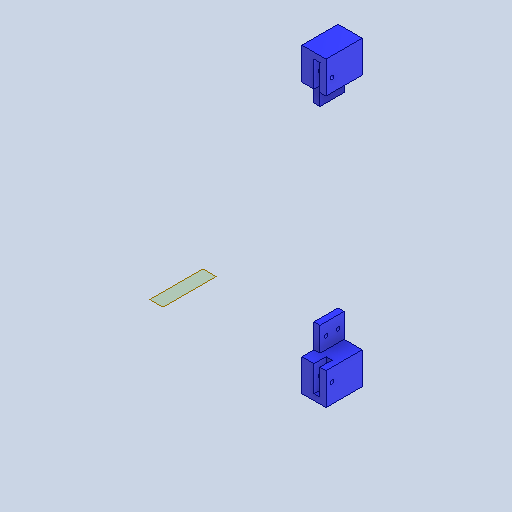
# Autodesk Inventor part: base_weel-v3-3DP-2
Saved by Autodesk Inventor 2025.2 (Build 292293000, 293)
## iProperties
Created: 2025-04-04
Part Number: base_weel-v3-3DP-2
Material: ABS プラスチック
Document SubType Name: Modeling
Designer: haruy
Density: 1.06 g/cm^3
Appearance: 青 - 壁塗料 - 光沢
Author: haruy
Autodesk Inventor part; units mm, degrees
ref_plane "YZ Plane" through (0, 0, 0) normal (1, 0, 0) x (0, 1, 0)
ref_plane "XZ Plane" through (0, 0, 0) normal (0, 1, 0) x (-1, 0, 0)
ref_plane "XY Plane" through (0, 0, 0) normal (0, 0, 1) x (1, 0, 0)
derived "base_weel-v3-3DP-1.ipt"
sketch "スケッチ1" plane through (0, 0, 0) normal (1, 0, 0) x (0, 1, 0)
  circle A0 centre (0, 0) radius 385
  circle A1 centre (0, 0) radius 360
  line L0 (190, 300) -> (-190, 300)
  line L1 (-190, 300) -> (-190, 280)
  line L2 (-190, 280) -> (190, 280)
  line L3 (190, 280) -> (190, 300)
  line L4 (300, 190) -> (280, 190)
  line L5 (280, 190) -> (280, -190)
  line L6 (280, -190) -> (300, -190)
  line L7 (300, -190) -> (300, 190)
  line L8 (208.9645, 286.7462) -> (286.7462, 208.9645)
  line L9 (286.7462, 208.9645) -> (272.6041, 194.8223)
  line L10 (272.6041, 194.8223) -> (194.8223, 272.6041)
  line L11 (194.8223, 272.6041) -> (208.9645, 286.7462)
  line L12 (208.9645, 286.7462) -> (318.9645, 286.7462) construction
  line L13 (118.4548, 217.4497) -> (217.4497, 118.4548)
  line L14 (217.4497, 118.4548) -> (203.3076, 104.3127)
  line L15 (203.3076, 104.3127) -> (104.3127, 203.3076)
  line L16 (104.3127, 203.3076) -> (118.4548, 217.4497)
  line L17 (118.4548, 217.4497) -> (258.4548, 217.4497) construction
  line L18 (189.519, 263.7652) -> (263.7652, 189.519)
  line L19 (263.7652, 189.519) -> (235.481, 161.2348)
  line L20 (235.481, 161.2348) -> (161.2348, 235.481)
  line L21 (161.2348, 235.481) -> (189.519, 263.7652)
  line L22 (189.519, 263.7652) -> (294.519, 263.7652) construction
  line L23 (180.6802, 201.8934) -> (201.8934, 180.6802)
  line L24 (201.8934, 180.6802) -> (194.8223, 173.6091)
  line L25 (194.8223, 173.6091) -> (173.6091, 194.8223)
  line L26 (173.6091, 194.8223) -> (180.6802, 201.8934)
  line L27 (180.6802, 201.8934) -> (210.6802, 201.8934) construction
  line L28 (170.0736, 198.3579) -> (198.3579, 170.0736)
  line L29 (198.3579, 170.0736) -> (194.1152, 165.831)
  line L30 (194.1152, 165.831) -> (165.831, 194.1152)
  line L31 (165.831, 194.1152) -> (170.0736, 198.3579)
  line L32 (198.3579, 170.0736) -> (194.1152, 165.831)
  line L33 (194.1152, 165.831) -> (222.3995, 137.5467)
  line L34 (222.3995, 137.5467) -> (226.6421, 141.7893)
  line L35 (226.6421, 141.7893) -> (198.3579, 170.0736)
  line L36 (197.6508, 162.2954) -> (218.864, 141.0822)
  line L37 (218.864, 141.0822) -> (211.7929, 134.0111)
  line L38 (211.7929, 134.0111) -> (190.5797, 155.2244)
  line L39 (190.5797, 155.2244) -> (197.6508, 162.2954)
  line L40 (182.448, 153.4566) -> (215.682, 120.2226)
  line L41 (215.682, 120.2226) -> (146.032, 50.5725)
  line L42 (146.032, 50.5725) -> (112.7979, 83.8066)
  line L43 (112.7979, 83.8066) -> (182.448, 153.4566)
  line L44 (193.4081, 142.4964) -> (199.065, 136.8396)
  line L45 (199.065, 136.8396) -> (215.5406, 153.3152)
  line L46 (215.5406, 153.3152) -> (209.8837, 158.972)
  line L47 (209.8837, 158.972) -> (193.4081, 142.4964)
  line L48 (58.5, 280) -> (38.5, 280)
  line L49 (38.5, 280) -> (38.5, -280)
  line L50 (38.5, -280) -> (58.5, -280)
  line L51 (58.5, -280) -> (58.5, 280)
  line L52 (280, 98.5) -> (58.5, 98.5)
  line L53 (58.5, 98.5) -> (58.5, 78.5)
  line L54 (58.5, 78.5) -> (280, 78.5)
  line L55 (280, 78.5) -> (280, 98.5)
  line L56 (156.5, 23.5) -> (58.5, 23.5)
  line L57 (58.5, 23.5) -> (58.5, -23.5)
  line L58 (58.5, -23.5) -> (156.5, -23.5)
  line L59 (156.5, -23.5) -> (156.5, 23.5)
  line L60 (98.5, 280) -> (78.5, 280)
  line L61 (78.5, 280) -> (78.5, 98.5)
  line L62 (78.5, 98.5) -> (98.5, 98.5)
  line L63 (98.5, 98.5) -> (98.5, 280)
  line L64 (23.5, 166.5) -> (-23.5, 166.5)
  line L65 (-23.5, 166.5) -> (-23.5, 68.5)
  line L66 (-23.5, 68.5) -> (23.5, 68.5)
  line L67 (23.5, 68.5) -> (23.5, 166.5)
  line L68 (-38.5, 280) -> (-58.5, 280)
  line L69 (-58.5, 280) -> (-58.5, -280)
  line L70 (-58.5, -280) -> (-38.5, -280)
  line L71 (-38.5, -280) -> (-38.5, 280)
  line L72 (23.5, -68.5) -> (-23.5, -68.5)
  line L73 (-23.5, -68.5) -> (-23.5, -166.5)
  line L74 (-23.5, -166.5) -> (23.5, -166.5)
  line L75 (23.5, -166.5) -> (23.5, -68.5)
  line L76 (-58.5, 23.5) -> (-156.5, 23.5)
  line L77 (-156.5, 23.5) -> (-156.5, -23.5)
  line L78 (-156.5, -23.5) -> (-58.5, -23.5)
  line L79 (-58.5, -23.5) -> (-58.5, 23.5)
  line L80 (-254.5584, -254.5584) -> (254.5584, -254.5584) construction
  line L81 (254.5584, -254.5584) -> (254.5584, 254.5584) construction
  line L82 (254.5584, 254.5584) -> (-254.5584, 254.5584) construction
  line L83 (-254.5584, 254.5584) -> (-254.5584, -254.5584) construction
  line L84 (-254.5584, -254.5584) -> (254.5584, 254.5584) construction
  line L85 (254.5584, -254.5584) -> (-254.5584, 254.5584) construction
  line L86 (254.5584, 254.5584) -> (0, 0)
  line L87 (0, 0) -> (0, 254.5584)
  line L88 (175.3769, 249.6231) -> (249.6231, 175.3769)
  line L89 (-212.5, -212.5) -> (212.5, -212.5) construction
  line L90 (212.5, -212.5) -> (212.5, 212.5) construction
  line L91 (212.5, 212.5) -> (-212.5, 212.5) construction
  line L92 (-212.5, 212.5) -> (-212.5, -212.5) construction
  line L93 (-212.5, -212.5) -> (212.5, 212.5) construction
  line L94 (212.5, -212.5) -> (-212.5, 212.5) construction
  line L95 (58.5, 68.5) -> (-58.5, 68.5)
  line L96 (-58.5, 68.5) -> (-58.5, 48.5)
  line L97 (-58.5, 48.5) -> (58.5, 48.5)
  line L98 (58.5, 48.5) -> (58.5, 68.5)
  line L99 (-58.5, -48.5) -> (58.5, -48.5)
  line L100 (58.5, -48.5) -> (58.5, -68.5)
  line L101 (58.5, -68.5) -> (-58.5, -68.5)
  line L102 (-58.5, -68.5) -> (-58.5, -48.5)
  line L103 (0, 0) -> (0, 300)
  line L104 (0, 0) -> (300, 0)
  line L105 (190, -300) -> (-190, -300)
  line L106 (-190, -300) -> (-190, -280)
  line L107 (-190, -280) -> (190, -280)
  line L108 (190, -280) -> (190, -300)
  line L109 (280, -98.5) -> (58.5, -98.5)
  line L110 (58.5, -78.5) -> (280, -78.5)
  line L111 (78.5, -280) -> (78.5, -98.5)
  line L112 (98.5, -98.5) -> (98.5, -280)
  line L113 (208.9645, -286.7462) -> (286.7462, -208.9645)
  line L114 (286.7462, -208.9645) -> (272.6041, -194.8223)
  line L115 (272.6041, -194.8223) -> (194.8223, -272.6041)
  line L116 (194.8223, -272.6041) -> (208.9645, -286.7462)
  line L117 (118.4548, -217.4497) -> (217.4497, -118.4548)
  line L118 (217.4497, -118.4548) -> (203.3076, -104.3127)
  line L119 (203.3076, -104.3127) -> (104.3127, -203.3076)
  line L120 (104.3127, -203.3076) -> (118.4548, -217.4497)
  line L121 (-300, 190) -> (-280, 190)
  line L122 (-280, 190) -> (-280, -190)
  line L123 (-280, -190) -> (-300, -190)
  line L124 (-300, -190) -> (-300, 190)
  line L125 (-208.9645, 286.7462) -> (-286.7462, 208.9645)
  line L126 (-286.7462, 208.9645) -> (-272.6041, 194.8223)
  line L127 (-272.6041, 194.8223) -> (-194.8223, 272.6041)
  line L128 (-194.8223, 272.6041) -> (-208.9645, 286.7462)
  line L129 (-118.4548, 217.4497) -> (-217.4497, 118.4548)
  line L130 (-217.4497, 118.4548) -> (-203.3076, 104.3127)
  line L131 (-203.3076, 104.3127) -> (-104.3127, 203.3076)
  line L132 (-104.3127, 203.3076) -> (-118.4548, 217.4497)
  line L133 (-280, 98.5) -> (-58.5, 98.5)
  line L134 (-58.5, 78.5) -> (-280, 78.5)
  line L135 (-78.5, 280) -> (-78.5, 98.5)
  line L136 (-98.5, 98.5) -> (-98.5, 280)
  line L137 (-98.5, -98.5) -> (-98.5, -280)
  line L138 (-78.5, -280) -> (-78.5, -98.5)
  line L139 (-280, -98.5) -> (-58.5, -98.5)
  line L140 (-58.5, -78.5) -> (-280, -78.5)
  line L141 (-208.9645, -286.7462) -> (-286.7462, -208.9645)
  line L142 (-194.8223, -272.6041) -> (-208.9645, -286.7462)
  line L143 (-272.6041, -194.8223) -> (-194.8223, -272.6041)
  line L144 (-286.7462, -208.9645) -> (-272.6041, -194.8223)
  line L145 (-118.4548, -217.4497) -> (-217.4497, -118.4548)
  line L146 (-104.3127, -203.3076) -> (-118.4548, -217.4497)
  line L147 (-203.3076, -104.3127) -> (-104.3127, -203.3076)
  line L148 (-217.4497, -118.4548) -> (-203.3076, -104.3127)
  line L149 (170, 300) -> (170, 280)
  line L150 (223.1066, 272.6041) -> (208.9645, 258.4619)
  circle A2 centre (175, 290) radius 1.6
  circle A3 centre (185, 290) radius 1.6
  circle A4 centre (205.4289, 276.1396) radius 1.6
  circle A5 centre (212.5, 269.0685) radius 1.6
  circle A6 centre (290, 175) radius 1.6
  circle A7 centre (290, 185) radius 1.6
  circle A8 centre (276.1396, 205.4289) radius 1.6
  circle A9 centre (269.0685, 212.5) radius 1.6
  line L151 (132.5969, 203.3076) -> (118.4548, 189.1655)
  line L152 (118.4548, 217.4497) -> (98.5, 237.4045)
  line L153 (104.3127, 203.3076) -> (98.5, 209.1203)
  line L154 (98.5, 209.1203) -> (78.5, 209.1203)
  circle A10 centre (88.5, 218) radius 1.6
  circle A11 centre (88.5, 228) radius 1.6
  line L155 (98.5, 237.4045) -> (78.5, 237.4045)
  circle A12 centre (121.9903, 199.7721) radius 1.6
  circle A13 centre (114.9193, 206.8431) radius 1.6
  circle A14 centre (218, 88.5) radius 1.6
  circle A15 centre (228, 88.5) radius 1.6
  circle A16 centre (199.7721, 121.9903) radius 1.6
  circle A17 centre (206.8431, 114.9193) radius 1.6
  line L156 (38.5, 280) -> (38.5, 300)
  line L157 (98.5, 280) -> (98.5, 300)
  line L158 (58.5, 260) -> (38.5, 260)
  line L159 (78.5, 260) -> (98.5, 260)
  circle A18 centre (88.5, 275) radius 1.6
  circle A19 centre (88.5, 265) radius 1.6
  circle A20 centre (48.5, 275) radius 1.6
  circle A21 centre (48.5, 265) radius 1.6
  circle A22 centre (88.5, 290) radius 1.6
  circle A23 centre (68.5, 290) radius 1.6
  circle A24 centre (48.5, 290) radius 1.6
  line L160 (260, 98.5) -> (260, 78.5)
  line L161 (300, 98.5) -> (280, 98.5)
  line L162 (280, 78.5) -> (300, 78.5)
  circle A25 centre (290, 78.5) radius 1.6
  circle A26 centre (290, 88.5) radius 1.6
  circle A27 centre (275, 88.5) radius 1.6
  circle A28 centre (265, 88.5) radius 1.6
  line L163 (78.5, 189.25) -> (58.5, 189.25)
  circle A29 centre (88.5, 103.5) radius 1.6
  circle A30 centre (88.5, 113.5) radius 1.6
  circle A31 centre (48.5, 103.5) radius 1.6
  circle A32 centre (48.5, 113.5) radius 1.6
  circle A33 centre (88.5, 88.5) radius 1.6
  circle A34 centre (68.5, 88.5) radius 1.6
  circle A35 centre (48.5, 88.5) radius 1.6
  circle A36 centre (48.5, 58.5) radius 1.6
  circle A37 centre (175, -290) radius 1.6
  circle A38 centre (185, -290) radius 1.6
  circle A39 centre (205.4289, -276.1396) radius 1.6
  circle A40 centre (212.5, -269.0685) radius 1.6
  circle A41 centre (276.1396, -205.4289) radius 1.6
  circle A42 centre (269.0685, -212.5) radius 1.6
  circle A43 centre (290, -185) radius 1.6
  circle A44 centre (290, -175) radius 1.6
  circle A45 centre (88.5, -218) radius 1.6
  circle A46 centre (88.5, -228) radius 1.6
  circle A47 centre (121.9903, -199.7721) radius 1.6
  circle A48 centre (114.9193, -206.8431) radius 1.6
  circle A49 centre (228, -88.5) radius 1.6
  circle A50 centre (218, -88.5) radius 1.6
  circle A51 centre (206.8431, -114.9193) radius 1.6
  circle A52 centre (199.7721, -121.9903) radius 1.6
  circle A53 centre (88.5, -275) radius 1.6
  circle A54 centre (88.5, -265) radius 1.6
  circle A55 centre (48.5, -275) radius 1.6
  circle A56 centre (48.5, -265) radius 1.6
  circle A57 centre (88.5, -290) radius 1.6
  circle A58 centre (68.5, -290) radius 1.6
  circle A59 centre (48.5, -290) radius 1.6
  circle A60 centre (290, -78.5) radius 1.6
  circle A61 centre (290, -88.5) radius 1.6
  circle A62 centre (275, -88.5) radius 1.6
  circle A63 centre (265, -88.5) radius 1.6
  circle A64 centre (88.5, -88.5) radius 1.6
  circle A65 centre (68.5, -88.5) radius 1.6
  circle A66 centre (48.5, -88.5) radius 1.6
  circle A67 centre (48.5, -103.5) radius 1.6
  circle A68 centre (48.5, -113.5) radius 1.6
  circle A69 centre (88.5, -103.5) radius 1.6
  circle A70 centre (88.5, -113.5) radius 1.6
  circle A71 centre (48.5, -58.5) radius 1.6
  circle A72 centre (-175, 290) radius 1.6
  circle A73 centre (-185, 290) radius 1.6
  circle A74 centre (-205.4289, 276.1396) radius 1.6
  circle A75 centre (-212.5, 269.0685) radius 1.6
  circle A76 centre (-276.1396, 205.4289) radius 1.6
  circle A77 centre (-269.0685, 212.5) radius 1.6
  circle A78 centre (-290, 185) radius 1.6
  circle A79 centre (-290, 175) radius 1.6
  circle A80 centre (-88.5, 218) radius 1.6
  circle A81 centre (-88.5, 228) radius 1.6
  circle A82 centre (-121.9903, 199.7721) radius 1.6
  circle A83 centre (-114.9193, 206.8431) radius 1.6
  circle A84 centre (-228, 88.5) radius 1.6
  circle A85 centre (-218, 88.5) radius 1.6
  circle A86 centre (-206.8431, 114.9193) radius 1.6
  circle A87 centre (-199.7721, 121.9903) radius 1.6
  circle A88 centre (-88.5, 275) radius 1.6
  circle A89 centre (-88.5, 265) radius 1.6
  circle A90 centre (-48.5, 275) radius 1.6
  circle A91 centre (-48.5, 265) radius 1.6
  circle A92 centre (-88.5, 290) radius 1.6
  circle A93 centre (-68.5, 290) radius 1.6
  circle A94 centre (-48.5, 290) radius 1.6
  circle A95 centre (-290, 78.5) radius 1.6
  circle A96 centre (-290, 88.5) radius 1.6
  circle A97 centre (-275, 88.5) radius 1.6
  circle A98 centre (-265, 88.5) radius 1.6
  circle A99 centre (-88.5, 88.5) radius 1.6
  circle A100 centre (-68.5, 88.5) radius 1.6
  circle A101 centre (-48.5, 88.5) radius 1.6
  circle A102 centre (-48.5, 103.5) radius 1.6
  circle A103 centre (-48.5, 113.5) radius 1.6
  circle A104 centre (-88.5, 103.5) radius 1.6
  circle A105 centre (-88.5, 113.5) radius 1.6
  circle A106 centre (-48.5, 58.5) radius 1.6
  circle A107 centre (-175, -290) radius 1.6
  circle A108 centre (-185, -290) radius 1.6
  circle A109 centre (-212.5, -269.0685) radius 1.6
  circle A110 centre (-205.4289, -276.1396) radius 1.6
  circle A111 centre (-269.0685, -212.5) radius 1.6
  circle A112 centre (-276.1396, -205.4289) radius 1.6
  circle A113 centre (-290, -185) radius 1.6
  circle A114 centre (-290, -175) radius 1.6
  circle A115 centre (-88.5, -290) radius 1.6
  circle A116 centre (-88.5, -275) radius 1.6
  circle A117 centre (-88.5, -265) radius 1.6
  circle A118 centre (-68.5, -290) radius 1.6
  circle A119 centre (-48.5, -290) radius 1.6
  circle A120 centre (-48.5, -275) radius 1.6
  circle A121 centre (-48.5, -265) radius 1.6
  circle A122 centre (-88.5, -228) radius 1.6
  circle A123 centre (-88.5, -218) radius 1.6
  circle A124 centre (-114.9193, -206.8431) radius 1.6
  circle A125 centre (-121.9903, -199.7721) radius 1.6
  circle A126 centre (-88.5, -113.5) radius 1.6
  circle A127 centre (-88.5, -103.5) radius 1.6
  circle A128 centre (-88.5, -88.5) radius 1.6
  circle A129 centre (-68.5, -88.5) radius 1.6
  circle A130 centre (-48.5, -88.5) radius 1.6
  circle A131 centre (-48.5, -103.5) radius 1.6
  circle A132 centre (-48.5, -113.5) radius 1.6
  circle A133 centre (-48.5, -58.5) radius 1.6
  circle A134 centre (-199.7721, -121.9903) radius 1.6
  circle A135 centre (-206.8431, -114.9193) radius 1.6
  circle A136 centre (-218, -88.5) radius 1.6
  circle A137 centre (-228, -88.5) radius 1.6
  circle A138 centre (-265, -88.5) radius 1.6
  circle A139 centre (-275, -88.5) radius 1.6
  circle A140 centre (-290, -78.5) radius 1.6
  circle A141 centre (-290, -88.5) radius 1.6
  line L164 (120, 280) -> (-120, 280)
  line L165 (-120, 280) -> (-120, 171.5)
  line L166 (-120, 171.5) -> (120, 171.5)
  line L167 (120, 171.5) -> (120, 280)
  line L168 (105, 300) -> (125, 300)
  line L169 (125, 300) -> (125, 280)
  line L170 (125, 280) -> (105, 280)
  line L171 (105, 280) -> (105, 300)
  line L172 (78.5, 171.5) -> (98.5, 171.5)
  line L173 (98.5, 171.5) -> (98.5, 151.5)
  line L174 (98.5, 151.5) -> (78.5, 151.5)
  line L175 (78.5, 151.5) -> (78.5, 171.5)
  circle A142 centre (120, 290) radius 1.6
  circle A143 centre (110, 290) radius 1.6
  circle A144 centre (88.5, 166.5) radius 1.6
  circle A145 centre (88.5, 156.5) radius 1.6
  circle A146 centre (-120, 290) radius 1.6
  circle A147 centre (-110, 290) radius 1.6
  circle A148 centre (-88.5, 166.5) radius 1.6
  circle A149 centre (-88.5, 156.5) radius 1.6
  circle A150 centre (120, -290) radius 1.6
  circle A151 centre (110, -290) radius 1.6
  circle A152 centre (88.5, -166.5) radius 1.6
  circle A153 centre (88.5, -156.5) radius 1.6
  circle A154 centre (-120, -290) radius 1.6
  circle A155 centre (-110, -290) radius 1.6
  circle A156 centre (-88.5, -166.5) radius 1.6
  circle A157 centre (-88.5, -156.5) radius 1.6
  line L176 (300, 73.5) -> (280, 73.5)
  circle A158 centre (290, 120) radius 1.6
  circle A159 centre (290, 110) radius 1.6
  circle A160 centre (166.5, 88.5) radius 1.6
  circle A161 centre (156.5, 88.5) radius 1.6
  circle A162 centre (290, -110) radius 1.6
  circle A163 centre (290, -120) radius 1.6
  circle A164 centre (166.5, -88.5) radius 1.6
  circle A165 centre (156.5, -88.5) radius 1.6
  line L177 (-161.5, 84) -> (-268.5, 84)
  line L178 (-268.5, 84) -> (-268.5, -84)
  line L179 (-268.5, -84) -> (-161.5, -84)
  line L180 (-161.5, -84) -> (-161.5, 84)
  circle A166 centre (-190.5, 35) radius 1.6
  circle A167 centre (-190.5, -35) radius 1.6
  circle A168 centre (-231, 35) radius 1.6
  circle A169 centre (-231, -35) radius 1.6
  line L181 (-200.5, 78.5) -> (-180.5, 78.5)
  line L182 (-180.5, 78.5) -> (-180.5, -78.5)
  line L183 (-180.5, -78.5) -> (-200.5, -78.5)
  line L184 (-200.5, -78.5) -> (-200.5, 78.5)
  line L185 (-241, 78.5) -> (-221, 78.5)
  line L186 (-221, 78.5) -> (-221, -78.5)
  line L187 (-221, -78.5) -> (-241, -78.5)
  line L188 (-241, -78.5) -> (-241, 78.5)
  line L189 (-180.5, 45) -> (-241, 45)
  line L190 (-180.5, -45) -> (-241, -45)
  line L191 (-221, 58.5) -> (-241, 58.5)
  line L192 (-180.5, 58.5) -> (-200.5, 58.5)
  circle A170 centre (-190.5, 73.5) radius 1.6
  circle A171 centre (-190.5, 63.5) radius 1.6
  circle A172 centre (-231, 73.5) radius 1.6
  circle A173 centre (-231, 63.5) radius 1.6
  circle A174 centre (-190.5, -73.5) radius 1.6
  circle A175 centre (-190.5, -63.5) radius 1.6
  circle A176 centre (-231, -73.5) radius 1.6
  circle A177 centre (-231, -63.5) radius 1.6
  line L193 (125, 280) -> (105, 280)
  line L194 (105, 280) -> (105, 260)
  line L195 (105, 260) -> (125, 260)
  line L196 (125, 260) -> (125, 280)
  line L197 (98.5, 151.5) -> (125, 151.5)
  line L198 (125, 151.5) -> (125, 181.5)
  line L199 (125, 181.5) -> (98.5, 181.5)
  line L200 (98.5, 181.5) -> (98.5, 151.5)
  circle A178 centre (112.5, 270) radius 1.6
  circle A179 centre (109.25, 176.5) radius 1.6
  point P0 (167.9523, 196.2365)
  point P1 (160, 290)
  point P2 (88.5, 280)
  point P3 (98.5, 171.5)
  point P4 (120, 181.5)
  dimension "d1" = 3.2
  dimension "d2" = 5
  dimension "d3" = 21.5
  dimension "d4" = 10.75
  measures "d1" diameter of A179
  measures "d2" distance from line of A179.centre L199
  measures "d3" distance between parallel lines of L200 L167
  measures "d4" distance from line of A179.centre L167
ref_plane "作業平面1" through (-5, 0, 300) normal (0, -1, 0) x (1, 0, 0)
extrude "押し出し1" add sketch "スケッチ1" along normal blind 5 contours L199 L167 L166 L63 | L199 L198 L197 L63 L166 L167 | L166 L63 L174 L61
extrude "押し出し2" add sketch "スケッチ1" along normal blind 5 from surface at 5 contours L199 L167 L166 L63 | L199 L198 L197 L63 L166 L167
extrude "押し出し3" add sketch "スケッチ1" along normal blind 5 from surface at 10 contours L199 L198 L197 L63 L166 L167
extrude "押し出し4" add sketch "スケッチ1" along normal blind 5 from surface at 15 contours L199 L167 L166 L63 | L199 L198 L197 L63 L166 L167
mirror "ミラー1" about plane through (-5, 0, 300) normal (0, -1, 0)
equation "\"d4\" = 0.5 * d3"
